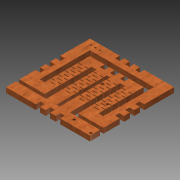
# Autodesk Inventor part: mech
Saved by Autodesk Inventor 2014 SP1 (Build 180222100, 222)
## iProperties
Created: 2015-02-17
Part Number: mech
Material: Wood (Cherry)
Document SubType Name: Modeling
Designer: Erin
Density: 0.63 g/cm^3
Appearance: Cherry - Natural Low Gloss
Author: Erin
Autodesk Inventor part; units mm, degrees
(part 1 of 2)
ref_plane "YZ Plane" through (0, 0, 0) normal (1, 0, 0) x (0, 1, 0)
ref_plane "XZ Plane" through (0, 0, 0) normal (0, 1, 0) x (-1, 0, 0)
ref_plane "XY Plane" through (0, 0, 0) normal (0, 0, 1) x (1, 0, 0)
sketch "slots" plane through (0, 0, 0) normal (0, 0, 1) x (1, 0, 0)
  line L0 (61.2067, 31.1821) -> (64.2567, 31.1821)
  line L1 (64.2567, 31.1821) -> (64.2567, 28.1071)
  line L2 (64.2567, 28.1071) -> (61.2067, 28.1071)
  line L3 (61.2067, 28.1071) -> (61.2067, 31.1821)
  line L4 (68.9317, 33.8834) -> (68.9317, 26.9198) construction
  line L5 (67.4067, 31.1821) -> (70.4567, 31.1821)
  line L6 (70.4567, 31.1821) -> (70.4567, 28.1071)
  line L7 (70.4567, 28.1071) -> (67.4067, 28.1071)
  line L8 (67.4067, 28.1071) -> (67.4067, 31.1821)
  line L9 (73.6067, 31.1821) -> (76.6567, 31.1821)
  line L10 (76.6567, 31.1821) -> (76.6567, 28.1071)
  line L11 (76.6567, 28.1071) -> (73.6067, 28.1071)
  line L12 (73.6067, 28.1071) -> (73.6067, 31.1821)
  line L13 (68.9317, 28.1071) -> (68.9317, 27.1937) construction
  point P0 (68.8645, 30.3856)
  dimension "d2" = 3.05
  dimension "d3" = 3.075
  dimension "d99" = 3.15
  dimension "d100" = 3.15
  measures "d2" distance of L1.end L2.end
  measures "d3" distance of L0.end L1.end
  measures "d99" distance between parallel lines of L8 L1
  measures "d100" distance between parallel lines of L12 L6
sketch "flexure" plane through (0, 0, 0) normal (0, 0, 1) x (1, 0, 0)
  line L0 (49.9032, 41.5133) -> (55.9032, 41.5133)
  line L1 (55.9032, 41.5133) -> (55.9032, 19.5133)
  line L2 (55.9032, 19.5133) -> (49.9032, 19.5133)
  line L3 (49.9032, 19.5133) -> (49.9032, 41.5133)
  line L4 (49.9032, 31.7633) -> (52.085, 31.7633)
  line L5 (52.085, 31.7633) -> (52.085, 31.2633)
  line L6 (52.085, 31.2633) -> (49.9032, 31.2633)
  line L7 (49.9032, 31.2633) -> (49.9032, 31.7633)
  line L8 (53.7214, 31.2633) -> (53.7214, 31.7633)
  line L9 (55.9032, 31.2633) -> (53.7214, 31.2633)
  line L10 (53.7214, 31.7633) -> (55.9032, 31.7633)
  line L11 (55.9032, 31.7633) -> (55.9032, 31.2633)
  line L12 (51.5395, 29.7633) -> (54.2668, 29.7633)
  line L13 (54.2668, 29.7633) -> (54.2668, 29.2633)
  line L14 (54.2668, 29.2633) -> (51.5395, 29.2633)
  line L15 (51.5395, 29.2633) -> (51.5395, 29.7633)
  line L16 (49.9032, 30.5133) -> (55.9032, 30.5133) construction
  line L17 (55.9032, 30.5133) -> (49.9032, 30.5133) construction
  line L18 (53.7214, 27.7633) -> (55.9032, 27.7633)
  line L19 (55.9032, 27.7633) -> (55.9032, 27.2633)
  line L20 (55.9032, 27.2633) -> (53.7214, 27.2633)
  line L21 (53.7214, 27.2633) -> (53.7214, 27.7633)
  line L22 (51.5395, 25.7633) -> (54.2668, 25.7633)
  line L23 (54.2668, 25.7633) -> (54.2668, 25.2633)
  line L24 (54.2668, 25.2633) -> (51.5395, 25.2633)
  line L25 (51.5395, 25.2633) -> (51.5395, 25.7633)
  line L26 (49.9032, 27.7633) -> (52.085, 27.7633)
  line L27 (52.085, 27.7633) -> (52.085, 27.2633)
  line L28 (52.085, 27.2633) -> (49.9032, 27.2633)
  line L29 (49.9032, 27.2633) -> (49.9032, 27.7633)
  line L30 (49.9032, 26.5133) -> (55.9032, 26.5133) construction
  line L31 (55.9032, 26.5133) -> (49.9032, 26.5133) construction
  line L32 (53.7214, 23.7633) -> (55.9032, 23.7633)
  line L33 (55.9032, 23.7633) -> (55.9032, 23.2633)
  line L34 (55.9032, 23.2633) -> (53.7214, 23.2633)
  line L35 (53.7214, 23.2633) -> (53.7214, 23.7633)
  line L36 (51.5395, 21.7633) -> (54.2668, 21.7633)
  line L37 (54.2668, 21.7633) -> (54.2668, 21.2633)
  line L38 (54.2668, 21.2633) -> (51.5395, 21.2633)
  line L39 (51.5395, 21.2633) -> (51.5395, 21.7633)
  line L40 (49.9032, 23.7633) -> (52.085, 23.7633)
  line L41 (52.085, 23.7633) -> (52.085, 23.2633)
  line L42 (52.085, 23.2633) -> (49.9032, 23.2633)
  line L43 (49.9032, 23.2633) -> (49.9032, 23.7633)
  line L44 (49.9032, 22.5133) -> (55.9032, 22.5133) construction
  line L45 (55.9032, 22.5133) -> (49.9032, 22.5133) construction
  line L46 (53.7214, 35.7633) -> (55.9032, 35.7633)
  line L47 (55.9032, 35.7633) -> (55.9032, 35.2633)
  line L48 (55.9032, 35.2633) -> (53.7214, 35.2633)
  line L49 (53.7214, 35.2633) -> (53.7214, 35.7633)
  line L50 (51.5395, 33.7633) -> (54.2668, 33.7633)
  line L51 (54.2668, 33.7633) -> (54.2668, 33.2633)
  line L52 (54.2668, 33.2633) -> (51.5395, 33.2633)
  line L53 (51.5395, 33.2633) -> (51.5395, 33.7633)
  line L54 (49.9032, 35.7633) -> (52.085, 35.7633)
  line L55 (52.085, 35.7633) -> (52.085, 35.2633)
  line L56 (52.085, 35.2633) -> (49.9032, 35.2633)
  line L57 (49.9032, 35.2633) -> (49.9032, 35.7633)
  line L58 (49.9032, 34.5133) -> (55.9032, 34.5133) construction
  line L59 (55.9032, 34.5133) -> (49.9032, 34.5133) construction
  line L60 (53.7214, 31.7633) -> (55.9032, 31.7633)
  line L61 (55.9032, 31.7633) -> (55.9032, 31.2633)
  line L62 (55.9032, 31.2633) -> (53.7214, 31.2633)
  line L63 (53.7214, 31.2633) -> (53.7214, 31.7633)
  line L64 (51.5395, 29.7633) -> (54.2668, 29.7633)
  line L65 (54.2668, 29.7633) -> (54.2668, 29.2633)
  line L66 (54.2668, 29.2633) -> (51.5395, 29.2633)
  line L67 (51.5395, 29.2633) -> (51.5395, 29.7633)
  line L68 (49.9032, 31.7633) -> (52.085, 31.7633)
  line L69 (52.085, 31.7633) -> (52.085, 31.2633)
  line L70 (52.085, 31.2633) -> (49.9032, 31.2633)
  line L71 (49.9032, 31.2633) -> (49.9032, 31.7633)
  line L72 (49.9032, 30.5133) -> (55.9032, 30.5133) construction
  line L73 (55.9032, 30.5133) -> (49.9032, 30.5133) construction
  line L74 (53.7214, 27.7633) -> (55.9032, 27.7633)
  line L75 (55.9032, 27.7633) -> (55.9032, 27.2633)
  line L76 (55.9032, 27.2633) -> (53.7214, 27.2633)
  line L77 (53.7214, 27.2633) -> (53.7214, 27.7633)
  line L78 (51.5395, 25.7633) -> (54.2668, 25.7633)
  line L79 (54.2668, 25.7633) -> (54.2668, 25.2633)
  line L80 (54.2668, 25.2633) -> (51.5395, 25.2633)
  line L81 (51.5395, 25.2633) -> (51.5395, 25.7633)
  line L82 (49.9032, 27.7633) -> (52.085, 27.7633)
  line L83 (52.085, 27.7633) -> (52.085, 27.2633)
  line L84 (52.085, 27.2633) -> (49.9032, 27.2633)
  line L85 (49.9032, 27.2633) -> (49.9032, 27.7633)
  line L86 (49.9032, 26.5133) -> (55.9032, 26.5133) construction
  line L87 (55.9032, 26.5133) -> (49.9032, 26.5133) construction
  line L88 (53.7214, 39.7633) -> (55.9032, 39.7633)
  line L89 (55.9032, 39.7633) -> (55.9032, 39.2633)
  line L90 (55.9032, 39.2633) -> (53.7214, 39.2633)
  line L91 (53.7214, 39.2633) -> (53.7214, 39.7633)
  line L92 (51.5395, 37.7633) -> (54.2668, 37.7633)
  line L93 (54.2668, 37.7633) -> (54.2668, 37.2633)
  line L94 (54.2668, 37.2633) -> (51.5395, 37.2633)
  line L95 (51.5395, 37.2633) -> (51.5395, 37.7633)
  line L96 (49.9032, 39.7633) -> (52.085, 39.7633)
  line L97 (52.085, 39.7633) -> (52.085, 39.2633)
  line L98 (52.085, 39.2633) -> (49.9032, 39.2633)
  line L99 (49.9032, 39.2633) -> (49.9032, 39.7633)
  line L100 (49.9032, 38.5133) -> (55.9032, 38.5133) construction
  line L101 (55.9032, 38.5133) -> (49.9032, 38.5133) construction
  line L102 (53.7214, 35.7633) -> (55.9032, 35.7633)
  line L103 (55.9032, 35.7633) -> (55.9032, 35.2633)
  line L104 (55.9032, 35.2633) -> (53.7214, 35.2633)
  line L105 (53.7214, 35.2633) -> (53.7214, 35.7633)
  line L106 (51.5395, 33.7633) -> (54.2668, 33.7633)
  line L107 (54.2668, 33.7633) -> (54.2668, 33.2633)
  line L108 (54.2668, 33.2633) -> (51.5395, 33.2633)
  line L109 (51.5395, 33.2633) -> (51.5395, 33.7633)
  line L110 (49.9032, 35.7633) -> (52.085, 35.7633)
  line L111 (52.085, 35.7633) -> (52.085, 35.2633)
  line L112 (52.085, 35.2633) -> (49.9032, 35.2633)
  line L113 (49.9032, 35.2633) -> (49.9032, 35.7633)
  line L114 (49.9032, 34.5133) -> (55.9032, 34.5133) construction
  line L115 (55.9032, 34.5133) -> (49.9032, 34.5133) construction
  line L116 (53.7214, 31.7633) -> (55.9032, 31.7633)
  line L117 (55.9032, 31.7633) -> (55.9032, 31.2633)
  line L118 (55.9032, 31.2633) -> (53.7214, 31.2633)
  line L119 (53.7214, 31.2633) -> (53.7214, 31.7633)
  line L120 (51.5395, 29.7633) -> (54.2668, 29.7633)
  line L121 (54.2668, 29.7633) -> (54.2668, 29.2633)
  line L122 (54.2668, 29.2633) -> (51.5395, 29.2633)
  line L123 (51.5395, 29.2633) -> (51.5395, 29.7633)
  line L124 (49.9032, 31.7633) -> (52.085, 31.7633)
  line L125 (52.085, 31.7633) -> (52.085, 31.2633)
  line L126 (52.085, 31.2633) -> (49.9032, 31.2633)
  line L127 (49.9032, 31.2633) -> (49.9032, 31.7633)
  line L128 (49.9032, 30.5133) -> (55.9032, 30.5133) construction
  line L129 (55.9032, 30.5133) -> (49.9032, 30.5133) construction
  line L130 (53.7214, 19.7633) -> (55.9032, 19.7633)
  line L131 (55.9032, 19.7633) -> (55.9032, 19.2633)
  line L132 (55.9032, 19.2633) -> (53.7214, 19.2633)
  line L133 (53.7214, 19.2633) -> (53.7214, 19.7633)
  line L134 (51.5395, 17.7633) -> (54.2668, 17.7633)
  line L135 (54.2668, 17.7633) -> (54.2668, 17.2633)
  line L136 (54.2668, 17.2633) -> (51.5395, 17.2633)
  line L137 (51.5395, 17.2633) -> (51.5395, 17.7633)
  line L138 (49.9032, 19.7633) -> (52.085, 19.7633)
  line L139 (52.085, 19.7633) -> (52.085, 19.2633)
  line L140 (52.085, 19.2633) -> (49.9032, 19.2633)
  line L141 (49.9032, 19.2633) -> (49.9032, 19.7633)
  line L142 (49.9032, 18.5133) -> (55.9032, 18.5133) construction
  line L143 (55.9032, 18.5133) -> (49.9032, 18.5133) construction
  line L144 (53.7214, 23.7633) -> (55.9032, 23.7633)
  line L145 (55.9032, 23.7633) -> (55.9032, 23.2633)
  line L146 (55.9032, 23.2633) -> (53.7214, 23.2633)
  line L147 (53.7214, 23.2633) -> (53.7214, 23.7633)
  line L148 (51.5395, 21.7633) -> (54.2668, 21.7633)
  line L149 (54.2668, 21.7633) -> (54.2668, 21.2633)
  line L150 (54.2668, 21.2633) -> (51.5395, 21.2633)
  line L151 (51.5395, 21.2633) -> (51.5395, 21.7633)
  line L152 (49.9032, 23.7633) -> (52.085, 23.7633)
  line L153 (52.085, 23.7633) -> (52.085, 23.2633)
  line L154 (52.085, 23.2633) -> (49.9032, 23.2633)
  line L155 (49.9032, 23.2633) -> (49.9032, 23.7633)
  line L156 (49.9032, 22.5133) -> (55.9032, 22.5133) construction
  line L157 (55.9032, 22.5133) -> (49.9032, 22.5133) construction
  line L158 (53.7214, 27.7633) -> (55.9032, 27.7633)
  line L159 (55.9032, 27.7633) -> (55.9032, 27.2633)
  line L160 (55.9032, 27.2633) -> (53.7214, 27.2633)
  line L161 (53.7214, 27.2633) -> (53.7214, 27.7633)
  line L162 (51.5395, 25.7633) -> (54.2668, 25.7633)
  line L163 (54.2668, 25.7633) -> (54.2668, 25.2633)
  line L164 (54.2668, 25.2633) -> (51.5395, 25.2633)
  line L165 (51.5395, 25.2633) -> (51.5395, 25.7633)
  line L166 (49.9032, 27.7633) -> (52.085, 27.7633)
  line L167 (52.085, 27.7633) -> (52.085, 27.2633)
  line L168 (52.085, 27.2633) -> (49.9032, 27.2633)
  line L169 (49.9032, 27.2633) -> (49.9032, 27.7633)
  line L170 (49.9032, 26.5133) -> (55.9032, 26.5133) construction
  line L171 (55.9032, 26.5133) -> (49.9032, 26.5133) construction
  line L172 (53.7214, 43.7633) -> (55.9032, 43.7633)
  line L173 (55.9032, 43.7633) -> (55.9032, 43.2633)
  line L174 (55.9032, 43.2633) -> (53.7214, 43.2633)
  line L175 (53.7214, 43.2633) -> (53.7214, 43.7633)
  line L176 (51.5395, 41.7633) -> (54.2668, 41.7633)
  line L177 (54.2668, 41.7633) -> (54.2668, 41.2633)
  line L178 (54.2668, 41.2633) -> (51.5395, 41.2633)
  line L179 (51.5395, 41.2633) -> (51.5395, 41.7633)
  line L180 (49.9032, 43.7633) -> (52.085, 43.7633)
  line L181 (52.085, 43.7633) -> (52.085, 43.2633)
  line L182 (52.085, 43.2633) -> (49.9032, 43.2633)
  line L183 (49.9032, 43.2633) -> (49.9032, 43.7633)
  line L184 (49.9032, 42.5133) -> (55.9032, 42.5133) construction
  line L185 (55.9032, 42.5133) -> (49.9032, 42.5133) construction
  line L186 (53.7214, 39.7633) -> (55.9032, 39.7633)
  line L187 (55.9032, 39.7633) -> (55.9032, 39.2633)
  line L188 (55.9032, 39.2633) -> (53.7214, 39.2633)
  line L189 (53.7214, 39.2633) -> (53.7214, 39.7633)
  line L190 (51.5395, 37.7633) -> (54.2668, 37.7633)
  line L191 (54.2668, 37.7633) -> (54.2668, 37.2633)
  line L192 (54.2668, 37.2633) -> (51.5395, 37.2633)
  line L193 (51.5395, 37.2633) -> (51.5395, 37.7633)
  line L194 (49.9032, 39.7633) -> (52.085, 39.7633)
  line L195 (52.085, 39.7633) -> (52.085, 39.2633)
  line L196 (52.085, 39.2633) -> (49.9032, 39.2633)
  line L197 (49.9032, 39.2633) -> (49.9032, 39.7633)
  line L198 (49.9032, 38.5133) -> (55.9032, 38.5133) construction
  line L199 (55.9032, 38.5133) -> (49.9032, 38.5133) construction
  line L200 (53.7214, 35.7633) -> (55.9032, 35.7633)
  line L201 (55.9032, 35.7633) -> (55.9032, 35.2633)
  line L202 (55.9032, 35.2633) -> (53.7214, 35.2633)
  line L203 (53.7214, 35.2633) -> (53.7214, 35.7633)
  line L204 (51.5395, 33.7633) -> (54.2668, 33.7633)
  line L205 (54.2668, 33.7633) -> (54.2668, 33.2633)
  line L206 (54.2668, 33.2633) -> (51.5395, 33.2633)
  line L207 (51.5395, 33.2633) -> (51.5395, 33.7633)
  line L208 (49.9032, 35.7633) -> (52.085, 35.7633)
  line L209 (52.085, 35.7633) -> (52.085, 35.2633)
  line L210 (52.085, 35.2633) -> (49.9032, 35.2633)
  line L211 (49.9032, 35.2633) -> (49.9032, 35.7633)
  line L212 (49.9032, 34.5133) -> (55.9032, 34.5133) construction
  line L213 (55.9032, 34.5133) -> (49.9032, 34.5133) construction
  line L214 (53.7214, 31.7633) -> (55.9032, 31.7633)
  line L215 (55.9032, 31.7633) -> (55.9032, 31.2633)
  line L216 (55.9032, 31.2633) -> (53.7214, 31.2633)
  line L217 (53.7214, 31.2633) -> (53.7214, 31.7633)
  line L218 (51.5395, 29.7633) -> (54.2668, 29.7633)
  line L219 (54.2668, 29.7633) -> (54.2668, 29.2633)
  line L220 (54.2668, 29.2633) -> (51.5395, 29.2633)
  line L221 (51.5395, 29.2633) -> (51.5395, 29.7633)
  line L222 (49.9032, 31.7633) -> (52.085, 31.7633)
  line L223 (52.085, 31.7633) -> (52.085, 31.2633)
  line L224 (52.085, 31.2633) -> (49.9032, 31.2633)
  line L225 (49.9032, 31.2633) -> (49.9032, 31.7633)
  line L226 (49.9032, 30.5133) -> (55.9032, 30.5133) construction
  line L227 (55.9032, 30.5133) -> (49.9032, 30.5133) construction
  point P0 (52.8239, 25.8216)
  dimension "d22" = 6
  dimension "d24" = 2.1818
  dimension "d27" = 3.8182
  dimension "d32" = 1.6364
  dimension "d33" = 2.7273
  dimension "d41" = 0.5
  dimension "d42" = 0.5
  dimension "d43" = 1.5
  dimension "d93" = 22
  dimension "d106" = 4
  dimension "d109" = 4
  dimension "d117" = 11.75
  measures "d22" distance of L1.end L2.end
  measures "d24" distance of L4.start L4.end
  measures "d27" distance of L6.end L9.end
  measures "d32" distance between parallel lines of L15 L3
  measures "d33" distance of L12.start L12.end
  measures "d41" distance of L4.end L5.end
  measures "d42" distance of L12.end L13.end
  measures "d43" distance between parallel lines of L12 L6
  measures "d93" distance of L0.end L1.end
  measures "d106" distance of L10.start L18.start
  measures "d109" distance of L10.start L46.start
  measures "d117" distance between parallel lines of L12 L0
sketch "Sketch1" plane through (0, 0, 0) normal (0, 0, 1) x (1, 0, 0)
  line L0 (-25, 25) -> (25, 25) construction
  line L1 (25, 25) -> (25, -25) construction
  line L2 (25, -25) -> (-25, -25) construction
  line L3 (-25, -25) -> (-25, 25) construction
  line L4 (-25, -25) -> (25, -25)
  line L5 (25, -25) -> (25, -19)
  line L6 (25, -19) -> (-25, -19)
  line L7 (-25, -19) -> (-25, -25)
  line L8 (0, 33.5916) -> (0, -39.9789) construction
  line L9 (-35.9054, 0) -> (42.6007, 0) construction
  line L10 (-25, 25) -> (25, 25)
  line L11 (25, 25) -> (25, 19)
  line L12 (25, 19) -> (-25, 19)
  line L13 (-25, 19) -> (-25, 25)
  line L14 (-25, 19) -> (-19, 19)
  line L15 (-19, 19) -> (-19, -17)
  line L16 (-19, -17) -> (-25, -17)
  line L17 (-25, -17) -> (-25, 19)
  line L18 (-19, -17) -> (-10, -17)
  line L19 (-10, -17) -> (-10, -11)
  line L20 (-10, -11) -> (-19, -11)
  line L21 (-19, -11) -> (-19, -17)
  line L22 (25, 19) -> (19, 19)
  line L23 (19, 19) -> (19, -17)
  line L24 (19, -17) -> (25, -17)
  line L25 (25, -17) -> (25, 19)
  line L26 (19, -17) -> (10, -17)
  line L27 (10, -17) -> (10, -11)
  line L28 (10, -11) -> (19, -11)
  line L29 (19, -11) -> (19, -17)
  line L30 (-16, 16) -> (16, 16)
  line L31 (16, 16) -> (16, 11)
  line L32 (16, 11) -> (-16, 11)
  line L33 (-16, 11) -> (-16, 16)
  line L34 (-7, -11) -> (-1, -11)
  line L35 (-1, -11) -> (-1, -19)
  line L36 (-1, -19) -> (-7, -19)
  line L37 (-7, -19) -> (-7, -11)
  line L38 (1, -11) -> (7, -11)
  line L39 (7, -11) -> (7, -19)
  line L40 (7, -19) -> (1, -19)
  line L41 (1, -19) -> (1, -11)
  line L42 (-68.1542, 16.5688) -> (-29.44, 16.5688) construction
  line L43 (-29.44, 16.5688) -> (-29.44, -5.0786) construction
  line L44 (-29.44, -5.0786) -> (-68.1542, -5.0786) construction
  line L45 (-68.1542, -5.0786) -> (-68.1542, 16.5688) construction
  circle A0 centre (-21.2866, 22) radius 0.5
  circle A1 centre (-18.6754, 22) radius 0.5
  circle A2 centre (-16, 22) radius 0.5
  line L46 (-7.725, 25) -> (-4.675, 25)
  line L47 (-4.675, 25) -> (-4.675, 21.925)
  line L48 (-4.675, 21.925) -> (-7.725, 21.925)
  line L49 (-7.725, 21.925) -> (-7.725, 25)
  line L50 (0, 27.7013) -> (0, 20.7377) construction
  line L51 (-1.525, 25) -> (1.525, 25)
  line L52 (1.525, 25) -> (1.525, 21.925)
  line L53 (1.525, 21.925) -> (-1.525, 21.925)
  line L54 (-1.525, 21.925) -> (-1.525, 25)
  line L55 (4.675, 25) -> (7.725, 25)
  line L56 (7.725, 25) -> (7.725, 21.925)
  line L57 (7.725, 21.925) -> (4.675, 21.925)
  line L58 (4.675, 21.925) -> (4.675, 25)
  line L59 (0, 21.925) -> (0, 21.0116) construction
  line L60 (-7.725, -21.925) -> (-4.675, -21.925)
  line L61 (-4.675, -21.925) -> (-4.675, -25)
  line L62 (-4.675, -25) -> (-7.725, -25)
  line L63 (-7.725, -25) -> (-7.725, -21.925)
  line L64 (0, -19.2237) -> (0, -26.1873) construction
  line L65 (-1.525, -21.925) -> (1.525, -21.925)
  line L66 (1.525, -21.925) -> (1.525, -25)
  line L67 (1.525, -25) -> (-1.525, -25)
  line L68 (-1.525, -25) -> (-1.525, -21.925)
  line L69 (4.675, -21.925) -> (7.725, -21.925)
  line L70 (7.725, -21.925) -> (7.725, -25)
  line L71 (7.725, -25) -> (4.675, -25)
  line L72 (4.675, -25) -> (4.675, -21.925)
  line L73 (0, -25) -> (0, -25.9134) construction
  line L74 (-25, -7.725) -> (-25, -4.675)
  line L75 (-25, -4.675) -> (-21.925, -4.675)
  line L76 (-21.925, -4.675) -> (-21.925, -7.725)
  line L77 (-21.925, -7.725) -> (-25, -7.725)
  line L78 (-27.7013, 0) -> (-20.7377, 0) construction
  line L79 (-25, -1.525) -> (-25, 1.525)
  line L80 (-25, 1.525) -> (-21.925, 1.525)
  line L81 (-21.925, 1.525) -> (-21.925, -1.525)
  line L82 (-21.925, -1.525) -> (-25, -1.525)
  line L83 (-25, 4.675) -> (-25, 7.725)
  line L84 (-25, 7.725) -> (-21.925, 7.725)
  line L85 (-21.925, 7.725) -> (-21.925, 4.675)
  line L86 (-21.925, 4.675) -> (-25, 4.675)
  line L87 (-21.925, 0) -> (-21.0116, 0) construction
  line L88 (21.925, -7.725) -> (21.925, -4.675)
  line L89 (21.925, -4.675) -> (25, -4.675)
  line L90 (25, -4.675) -> (25, -7.725)
  line L91 (25, -7.725) -> (21.925, -7.725)
  line L92 (19.2237, 0) -> (26.1873, 0) construction
  line L93 (21.925, -1.525) -> (21.925, 1.525)
  line L94 (21.925, 1.525) -> (25, 1.525)
  line L95 (25, 1.525) -> (25, -1.525)
  line L96 (25, -1.525) -> (21.925, -1.525)
  line L97 (21.925, 4.675) -> (21.925, 7.725)
  line L98 (21.925, 7.725) -> (25, 7.725)
  line L99 (25, 7.725) -> (25, 4.675)
  line L100 (25, 4.675) -> (21.925, 4.675)
  line L101 (25, 0) -> (25.9134, 0) construction
  line L102 (-16, 11) -> (-10, 11)
  line L103 (-10, 11) -> (-10, -11)
  line L104 (-10, -11) -> (-16, -11)
  line L105 (-16, -11) -> (-16, 11)
  line L106 (-16, 1.25) -> (-13.8182, 1.25)
  line L107 (-13.8182, 1.25) -> (-13.8182, 0.75)
  line L108 (-13.8182, 0.75) -> (-16, 0.75)
  line L109 (-16, 0.75) -> (-16, 1.25)
  line L110 (-12.1818, 0.75) -> (-12.1818, 1.25)
  line L111 (-10, 0.75) -> (-12.1818, 0.75)
  line L112 (-12.1818, 1.25) -> (-10, 1.25)
  line L113 (-10, 1.25) -> (-10, 0.75)
  line L114 (-14.3636, -0.75) -> (-11.6364, -0.75)
  line L115 (-11.6364, -0.75) -> (-11.6364, -1.25)
  line L116 (-11.6364, -1.25) -> (-14.3636, -1.25)
  line L117 (-14.3636, -1.25) -> (-14.3636, -0.75)
  line L118 (-16, 0) -> (-10, 0) construction
  line L119 (-10, 0) -> (-16, 0) construction
  line L120 (-12.1818, -2.75) -> (-10, -2.75)
  line L121 (-10, -2.75) -> (-10, -3.25)
  line L122 (-10, -3.25) -> (-12.1818, -3.25)
  line L123 (-12.1818, -3.25) -> (-12.1818, -2.75)
  line L124 (-14.3636, -4.75) -> (-11.6364, -4.75)
  line L125 (-11.6364, -4.75) -> (-11.6364, -5.25)
  line L126 (-11.6364, -5.25) -> (-14.3636, -5.25)
  line L127 (-14.3636, -5.25) -> (-14.3636, -4.75)
  line L128 (-16, -2.75) -> (-13.8182, -2.75)
  line L129 (-13.8182, -2.75) -> (-13.8182, -3.25)
  line L130 (-13.8182, -3.25) -> (-16, -3.25)
  line L131 (-16, -3.25) -> (-16, -2.75)
  line L132 (-16, -4) -> (-10, -4) construction
  line L133 (-10, -4) -> (-16, -4) construction
  line L134 (-12.1818, -6.75) -> (-10, -6.75)
  line L135 (-10, -6.75) -> (-10, -7.25)
  line L136 (-10, -7.25) -> (-12.1818, -7.25)
  line L137 (-12.1818, -7.25) -> (-12.1818, -6.75)
  line L138 (-14.3636, -8.75) -> (-11.6364, -8.75)
  line L139 (-11.6364, -8.75) -> (-11.6364, -9.25)
  line L140 (-11.6364, -9.25) -> (-14.3636, -9.25)
  line L141 (-14.3636, -9.25) -> (-14.3636, -8.75)
  line L142 (-16, -6.75) -> (-13.8182, -6.75)
  line L143 (-13.8182, -6.75) -> (-13.8182, -7.25)
  line L144 (-13.8182, -7.25) -> (-16, -7.25)
  line L145 (-16, -7.25) -> (-16, -6.75)
  line L146 (-16, -8) -> (-10, -8) construction
  line L147 (-10, -8) -> (-16, -8) construction
  line L148 (-12.1818, 5.25) -> (-10, 5.25)
  line L149 (-10, 5.25) -> (-10, 4.75)
  line L150 (-10, 4.75) -> (-12.1818, 4.75)
  line L151 (-12.1818, 4.75) -> (-12.1818, 5.25)
  line L152 (-14.3636, 3.25) -> (-11.6364, 3.25)
  line L153 (-11.6364, 3.25) -> (-11.6364, 2.75)
  line L154 (-11.6364, 2.75) -> (-14.3636, 2.75)
  line L155 (-14.3636, 2.75) -> (-14.3636, 3.25)
  line L156 (-16, 5.25) -> (-13.8182, 5.25)
  line L157 (-13.8182, 5.25) -> (-13.8182, 4.75)
  line L158 (-13.8182, 4.75) -> (-16, 4.75)
  line L159 (-16, 4.75) -> (-16, 5.25)
  line L160 (-16, 4) -> (-10, 4) construction
  line L161 (-10, 4) -> (-16, 4) construction
  line L162 (-12.1818, 1.25) -> (-10, 1.25)
  line L163 (-10, 1.25) -> (-10, 0.75)
  line L164 (-10, 0.75) -> (-12.1818, 0.75)
  line L165 (-12.1818, 0.75) -> (-12.1818, 1.25)
  line L166 (-14.3636, -0.75) -> (-11.6364, -0.75)
  line L167 (-11.6364, -0.75) -> (-11.6364, -1.25)
  line L168 (-11.6364, -1.25) -> (-14.3636, -1.25)
  line L169 (-14.3636, -1.25) -> (-14.3636, -0.75)
  line L170 (-16, 1.25) -> (-13.8182, 1.25)
  line L171 (-13.8182, 1.25) -> (-13.8182, 0.75)
  line L172 (-13.8182, 0.75) -> (-16, 0.75)
  line L173 (-16, 0.75) -> (-16, 1.25)
  line L174 (-16, 0) -> (-10, 0) construction
  line L175 (-10, 0) -> (-16, 0) construction
  line L176 (-12.1818, -2.75) -> (-10, -2.75)
  line L177 (-10, -2.75) -> (-10, -3.25)
  line L178 (-10, -3.25) -> (-12.1818, -3.25)
  line L179 (-12.1818, -3.25) -> (-12.1818, -2.75)
  line L180 (-14.3636, -4.75) -> (-11.6364, -4.75)
  line L181 (-11.6364, -4.75) -> (-11.6364, -5.25)
  line L182 (-11.6364, -5.25) -> (-14.3636, -5.25)
  line L183 (-14.3636, -5.25) -> (-14.3636, -4.75)
  line L184 (-16, -2.75) -> (-13.8182, -2.75)
  line L185 (-13.8182, -2.75) -> (-13.8182, -3.25)
  line L186 (-13.8182, -3.25) -> (-16, -3.25)
  line L187 (-16, -3.25) -> (-16, -2.75)
  line L188 (-16, -4) -> (-10, -4) construction
  line L189 (-10, -4) -> (-16, -4) construction
  line L190 (-12.1818, 9.25) -> (-10, 9.25)
  line L191 (-10, 9.25) -> (-10, 8.75)
  line L192 (-10, 8.75) -> (-12.1818, 8.75)
  line L193 (-12.1818, 8.75) -> (-12.1818, 9.25)
  line L194 (-14.3636, 7.25) -> (-11.6364, 7.25)
  line L195 (-11.6364, 7.25) -> (-11.6364, 6.75)
  line L196 (-11.6364, 6.75) -> (-14.3636, 6.75)
  line L197 (-14.3636, 6.75) -> (-14.3636, 7.25)
  line L198 (-16, 9.25) -> (-13.8182, 9.25)
  line L199 (-13.8182, 9.25) -> (-13.8182, 8.75)
  line L200 (-13.8182, 8.75) -> (-16, 8.75)
  line L201 (-16, 8.75) -> (-16, 9.25)
  line L202 (-16, 8) -> (-10, 8) construction
  line L203 (-10, 8) -> (-16, 8) construction
  line L204 (-12.1818, 5.25) -> (-10, 5.25)
  line L205 (-10, 5.25) -> (-10, 4.75)
  line L206 (-10, 4.75) -> (-12.1818, 4.75)
  line L207 (-12.1818, 4.75) -> (-12.1818, 5.25)
  line L208 (-14.3636, 3.25) -> (-11.6364, 3.25)
  line L209 (-11.6364, 3.25) -> (-11.6364, 2.75)
  line L210 (-11.6364, 2.75) -> (-14.3636, 2.75)
  line L211 (-14.3636, 2.75) -> (-14.3636, 3.25)
  line L212 (-16, 5.25) -> (-13.8182, 5.25)
  line L213 (-13.8182, 5.25) -> (-13.8182, 4.75)
  line L214 (-13.8182, 4.75) -> (-16, 4.75)
  line L215 (-16, 4.75) -> (-16, 5.25)
  line L216 (-16, 4) -> (-10, 4) construction
  line L217 (-10, 4) -> (-16, 4) construction
  line L218 (-12.1818, 1.25) -> (-10, 1.25)
  line L219 (-10, 1.25) -> (-10, 0.75)
  line L220 (-10, 0.75) -> (-12.1818, 0.75)
  line L221 (-12.1818, 0.75) -> (-12.1818, 1.25)
  line L222 (-14.3636, -0.75) -> (-11.6364, -0.75)
  line L223 (-11.6364, -0.75) -> (-11.6364, -1.25)
  line L224 (-11.6364, -1.25) -> (-14.3636, -1.25)
  line L225 (-14.3636, -1.25) -> (-14.3636, -0.75)
  line L226 (-16, 1.25) -> (-13.8182, 1.25)
  line L227 (-13.8182, 1.25) -> (-13.8182, 0.75)
  line L228 (-13.8182, 0.75) -> (-16, 0.75)
  line L229 (-16, 0.75) -> (-16, 1.25)
  line L230 (-16, 0) -> (-10, 0) construction
  line L231 (-10, 0) -> (-16, 0) construction
  line L232 (-12.1818, -10.75) -> (-10, -10.75)
  line L233 (-10, -10.75) -> (-10, -11.25)
  line L234 (-10, -11.25) -> (-12.1818, -11.25)
  line L235 (-12.1818, -11.25) -> (-12.1818, -10.75)
  line L236 (-14.3636, -12.75) -> (-11.6364, -12.75)
  line L237 (-11.6364, -12.75) -> (-11.6364, -13.25)
  line L238 (-11.6364, -13.25) -> (-14.3636, -13.25)
  line L239 (-14.3636, -13.25) -> (-14.3636, -12.75)
  line L240 (-16, -10.75) -> (-13.8182, -10.75)
  line L241 (-13.8182, -10.75) -> (-13.8182, -11.25)
  line L242 (-13.8182, -11.25) -> (-16, -11.25)
  line L243 (-16, -11.25) -> (-16, -10.75)
  line L244 (-16, -12) -> (-10, -12) construction
  line L245 (-10, -12) -> (-16, -12) construction
  line L246 (-12.1818, -6.75) -> (-10, -6.75)
  line L247 (-10, -6.75) -> (-10, -7.25)
  line L248 (-10, -7.25) -> (-12.1818, -7.25)
  line L249 (-12.1818, -7.25) -> (-12.1818, -6.75)
  line L250 (-14.3636, -8.75) -> (-11.6364, -8.75)
  line L251 (-11.6364, -8.75) -> (-11.6364, -9.25)
  line L252 (-11.6364, -9.25) -> (-14.3636, -9.25)
  line L253 (-14.3636, -9.25) -> (-14.3636, -8.75)
  line L254 (-16, -6.75) -> (-13.8182, -6.75)
  line L255 (-13.8182, -6.75) -> (-13.8182, -7.25)
  line L256 (-13.8182, -7.25) -> (-16, -7.25)
  line L257 (-16, -7.25) -> (-16, -6.75)
  line L258 (-16, -8) -> (-10, -8) construction
  line L259 (-10, -8) -> (-16, -8) construction
  line L260 (-12.1818, -2.75) -> (-10, -2.75)
  line L261 (-10, -2.75) -> (-10, -3.25)
  line L262 (-10, -3.25) -> (-12.1818, -3.25)
  line L263 (-12.1818, -3.25) -> (-12.1818, -2.75)
  line L264 (-14.3636, -4.75) -> (-11.6364, -4.75)
  line L265 (-11.6364, -4.75) -> (-11.6364, -5.25)
  line L266 (-11.6364, -5.25) -> (-14.3636, -5.25)
  line L267 (-14.3636, -5.25) -> (-14.3636, -4.75)
  line L268 (-16, -2.75) -> (-13.8182, -2.75)
  line L269 (-13.8182, -2.75) -> (-13.8182, -3.25)
  line L270 (-13.8182, -3.25) -> (-16, -3.25)
  line L271 (-16, -3.25) -> (-16, -2.75)
  line L272 (-16, -4) -> (-10, -4) construction
  line L273 (-10, -4) -> (-16, -4) construction
  line L274 (-12.1818, 13.25) -> (-10, 13.25)
  line L275 (-10, 13.25) -> (-10, 12.75)
  line L276 (-10, 12.75) -> (-12.1818, 12.75)
  line L277 (-12.1818, 12.75) -> (-12.1818, 13.25)
  line L278 (-14.3636, 11.25) -> (-11.6364, 11.25)
  line L279 (-11.6364, 11.25) -> (-11.6364, 10.75)
  line L280 (-11.6364, 10.75) -> (-14.3636, 10.75)
  line L281 (-14.3636, 10.75) -> (-14.3636, 11.25)
  line L282 (-16, 13.25) -> (-13.8182, 13.25)
  line L283 (-13.8182, 13.25) -> (-13.8182, 12.75)
  line L284 (-13.8182, 12.75) -> (-16, 12.75)
  line L285 (-16, 12.75) -> (-16, 13.25)
  line L286 (-16, 12) -> (-10, 12) construction
  line L287 (-10, 12) -> (-16, 12) construction
  line L288 (-12.1818, 9.25) -> (-10, 9.25)
  line L289 (-10, 9.25) -> (-10, 8.75)
  line L290 (-10, 8.75) -> (-12.1818, 8.75)
  line L291 (-12.1818, 8.75) -> (-12.1818, 9.25)
  line L292 (-14.3636, 7.25) -> (-11.6364, 7.25)
  line L293 (-11.6364, 7.25) -> (-11.6364, 6.75)
  line L294 (-11.6364, 6.75) -> (-14.3636, 6.75)
  line L295 (-14.3636, 6.75) -> (-14.3636, 7.25)
  line L296 (-16, 9.25) -> (-13.8182, 9.25)
  line L297 (-13.8182, 9.25) -> (-13.8182, 8.75)
  line L298 (-13.8182, 8.75) -> (-16, 8.75)
  line L299 (-16, 8.75) -> (-16, 9.25)
  line L300 (-16, 8) -> (-10, 8) construction
  line L301 (-10, 8) -> (-16, 8) construction
  line L302 (-12.1818, 5.25) -> (-10, 5.25)
  line L303 (-10, 5.25) -> (-10, 4.75)
  line L304 (-10, 4.75) -> (-12.1818, 4.75)
  line L305 (-12.1818, 4.75) -> (-12.1818, 5.25)
  line L306 (-14.3636, 3.25) -> (-11.6364, 3.25)
  line L307 (-11.6364, 3.25) -> (-11.6364, 2.75)
  line L308 (-11.6364, 2.75) -> (-14.3636, 2.75)
  line L309 (-14.3636, 2.75) -> (-14.3636, 3.25)
  line L310 (-16, 5.25) -> (-13.8182, 5.25)
  line L311 (-13.8182, 5.25) -> (-13.8182, 4.75)
  line L312 (-13.8182, 4.75) -> (-16, 4.75)
  line L313 (-16, 4.75) -> (-16, 5.25)
  line L314 (-16, 4) -> (-10, 4) construction
  line L315 (-10, 4) -> (-16, 4) construction
  line L316 (-12.1818, 1.25) -> (-10, 1.25)
  line L317 (-10, 1.25) -> (-10, 0.75)
  line L318 (-10, 0.75) -> (-12.1818, 0.75)
  line L319 (-12.1818, 0.75) -> (-12.1818, 1.25)
  line L320 (-14.3636, -0.75) -> (-11.6364, -0.75)
  line L321 (-11.6364, -0.75) -> (-11.6364, -1.25)
  line L322 (-11.6364, -1.25) -> (-14.3636, -1.25)
  line L323 (-14.3636, -1.25) -> (-14.3636, -0.75)
  line L324 (-16, 1.25) -> (-13.8182, 1.25)
  line L325 (-13.8182, 1.25) -> (-13.8182, 0.75)
  line L326 (-13.8182, 0.75) -> (-16, 0.75)
  line L327 (-16, 0.75) -> (-16, 1.25)
  line L328 (-16, 0) -> (-10, 0) construction
  line L329 (-10, 0) -> (-16, 0) construction
  line L330 (10, 11) -> (16, 11)
  line L331 (16, 11) -> (16, -11)
  line L332 (16, -11) -> (10, -11)
  line L333 (10, -11) -> (10, 11)
  line L334 (10, 1.25) -> (12.1818, 1.25)
  line L335 (12.1818, 1.25) -> (12.1818, 0.75)
  line L336 (12.1818, 0.75) -> (10, 0.75)
  line L337 (10, 0.75) -> (10, 1.25)
  line L338 (13.8182, 0.75) -> (13.8182, 1.25)
  line L339 (16, 0.75) -> (13.8182, 0.75)
  line L340 (13.8182, 1.25) -> (16, 1.25)
  line L341 (16, 1.25) -> (16, 0.75)
  line L342 (11.6364, -0.75) -> (14.3636, -0.75)
  line L343 (14.3636, -0.75) -> (14.3636, -1.25)
  line L344 (14.3636, -1.25) -> (11.6364, -1.25)
  line L345 (11.6364, -1.25) -> (11.6364, -0.75)
  line L346 (10, 0) -> (16, 0) construction
  line L347 (16, 0) -> (10, 0) construction
  line L348 (13.8182, -2.75) -> (16, -2.75)
  line L349 (16, -2.75) -> (16, -3.25)
  line L350 (16, -3.25) -> (13.8182, -3.25)
  line L351 (13.8182, -3.25) -> (13.8182, -2.75)
  line L352 (11.6364, -4.75) -> (14.3636, -4.75)
  line L353 (14.3636, -4.75) -> (14.3636, -5.25)
  line L354 (14.3636, -5.25) -> (11.6364, -5.25)
  line L355 (11.6364, -5.25) -> (11.6364, -4.75)
  line L356 (10, -2.75) -> (12.1818, -2.75)
  line L357 (12.1818, -2.75) -> (12.1818, -3.25)
  line L358 (12.1818, -3.25) -> (10, -3.25)
  line L359 (10, -3.25) -> (10, -2.75)
  line L360 (10, -4) -> (16, -4) construction
  line L361 (16, -4) -> (10, -4) construction
  line L362 (13.8182, -6.75) -> (16, -6.75)
  line L363 (16, -6.75) -> (16, -7.25)
  line L364 (16, -7.25) -> (13.8182, -7.25)
  line L365 (13.8182, -7.25) -> (13.8182, -6.75)
  line L366 (11.6364, -8.75) -> (14.3636, -8.75)
  line L367 (14.3636, -8.75) -> (14.3636, -9.25)
  line L368 (14.3636, -9.25) -> (11.6364, -9.25)
  line L369 (11.6364, -9.25) -> (11.6364, -8.75)
  line L370 (10, -6.75) -> (12.1818, -6.75)
  line L371 (12.1818, -6.75) -> (12.1818, -7.25)
  line L372 (12.1818, -7.25) -> (10, -7.25)
  line L373 (10, -7.25) -> (10, -6.75)
  line L374 (10, -8) -> (16, -8) construction
  line L375 (16, -8) -> (10, -8) construction
  line L376 (13.8182, 5.25) -> (16, 5.25)
  line L377 (16, 5.25) -> (16, 4.75)
  line L378 (16, 4.75) -> (13.8182, 4.75)
  line L379 (13.8182, 4.75) -> (13.8182, 5.25)
  line L380 (11.6364, 3.25) -> (14.3636, 3.25)
  line L381 (14.3636, 3.25) -> (14.3636, 2.75)
  line L382 (14.3636, 2.75) -> (11.6364, 2.75)
  line L383 (11.6364, 2.75) -> (11.6364, 3.25)
  line L384 (10, 5.25) -> (12.1818, 5.25)
  line L385 (12.1818, 5.25) -> (12.1818, 4.75)
  line L386 (12.1818, 4.75) -> (10, 4.75)
  line L387 (10, 4.75) -> (10, 5.25)
  line L388 (10, 4) -> (16, 4) construction
  line L389 (16, 4) -> (10, 4) construction
  line L390 (13.8182, 1.25) -> (16, 1.25)
  line L391 (16, 1.25) -> (16, 0.75)
  line L392 (16, 0.75) -> (13.8182, 0.75)
  line L393 (13.8182, 0.75) -> (13.8182, 1.25)
  line L394 (11.6364, -0.75) -> (14.3636, -0.75)
  line L395 (14.3636, -0.75) -> (14.3636, -1.25)
  line L396 (14.3636, -1.25) -> (11.6364, -1.25)
  line L397 (11.6364, -1.25) -> (11.6364, -0.75)
  line L398 (10, 1.25) -> (12.1818, 1.25)
  line L399 (12.1818, 1.25) -> (12.1818, 0.75)
  line L400 (12.1818, 0.75) -> (10, 0.75)
  line L401 (10, 0.75) -> (10, 1.25)
  line L402 (10, 0) -> (16, 0) construction
  line L403 (16, 0) -> (10, 0) construction
  line L404 (13.8182, -2.75) -> (16, -2.75)
  line L405 (16, -2.75) -> (16, -3.25)
  line L406 (16, -3.25) -> (13.8182, -3.25)
  line L407 (13.8182, -3.25) -> (13.8182, -2.75)
  line L408 (11.6364, -4.75) -> (14.3636, -4.75)
  line L409 (14.3636, -4.75) -> (14.3636, -5.25)
  line L410 (14.3636, -5.25) -> (11.6364, -5.25)
  line L411 (11.6364, -5.25) -> (11.6364, -4.75)
  line L412 (10, -2.75) -> (12.1818, -2.75)
  line L413 (12.1818, -2.75) -> (12.1818, -3.25)
  line L414 (12.1818, -3.25) -> (10, -3.25)
  line L415 (10, -3.25) -> (10, -2.75)
  line L416 (10, -4) -> (16, -4) construction
  line L417 (16, -4) -> (10, -4) construction
  line L418 (13.8182, 9.25) -> (16, 9.25)
  line L419 (16, 9.25) -> (16, 8.75)
  line L420 (16, 8.75) -> (13.8182, 8.75)
  line L421 (13.8182, 8.75) -> (13.8182, 9.25)
  line L422 (11.6364, 7.25) -> (14.3636, 7.25)
  line L423 (14.3636, 7.25) -> (14.3636, 6.75)
  line L424 (14.3636, 6.75) -> (11.6364, 6.75)
  line L425 (11.6364, 6.75) -> (11.6364, 7.25)
  line L426 (10, 9.25) -> (12.1818, 9.25)
  line L427 (12.1818, 9.25) -> (12.1818, 8.75)
  line L428 (12.1818, 8.75) -> (10, 8.75)
  line L429 (10, 8.75) -> (10, 9.25)
  line L430 (10, 8) -> (16, 8) construction
  line L431 (16, 8) -> (10, 8) construction
  line L432 (13.8182, 5.25) -> (16, 5.25)
  line L433 (16, 5.25) -> (16, 4.75)
  line L434 (16, 4.75) -> (13.8182, 4.75)
  line L435 (13.8182, 4.75) -> (13.8182, 5.25)
  line L436 (11.6364, 3.25) -> (14.3636, 3.25)
  line L437 (14.3636, 3.25) -> (14.3636, 2.75)
  line L438 (14.3636, 2.75) -> (11.6364, 2.75)
  line L439 (11.6364, 2.75) -> (11.6364, 3.25)
  line L440 (10, 5.25) -> (12.1818, 5.25)
  line L441 (12.1818, 5.25) -> (12.1818, 4.75)
  line L442 (12.1818, 4.75) -> (10, 4.75)
  line L443 (10, 4.75) -> (10, 5.25)
  line L444 (10, 4) -> (16, 4) construction
  line L445 (16, 4) -> (10, 4) construction
  line L446 (13.8182, 1.25) -> (16, 1.25)
  line L447 (16, 1.25) -> (16, 0.75)
  line L448 (16, 0.75) -> (13.8182, 0.75)
  line L449 (13.8182, 0.75) -> (13.8182, 1.25)
  line L450 (11.6364, -0.75) -> (14.3636, -0.75)
  line L451 (14.3636, -0.75) -> (14.3636, -1.25)
  line L452 (14.3636, -1.25) -> (11.6364, -1.25)
  line L453 (11.6364, -1.25) -> (11.6364, -0.75)
  line L454 (10, 1.25) -> (12.1818, 1.25)
  line L455 (12.1818, 1.25) -> (12.1818, 0.75)
  line L456 (12.1818, 0.75) -> (10, 0.75)
  line L457 (10, 0.75) -> (10, 1.25)
  line L458 (10, 0) -> (16, 0) construction
  line L459 (16, 0) -> (10, 0) construction
  line L460 (13.8182, -10.75) -> (16, -10.75)
  line L461 (16, -10.75) -> (16, -11.25)
  line L462 (16, -11.25) -> (13.8182, -11.25)
  line L463 (13.8182, -11.25) -> (13.8182, -10.75)
  line L464 (11.6364, -12.75) -> (14.3636, -12.75)
  line L465 (14.3636, -12.75) -> (14.3636, -13.25)
  line L466 (14.3636, -13.25) -> (11.6364, -13.25)
  line L467 (11.6364, -13.25) -> (11.6364, -12.75)
  line L468 (10, -10.75) -> (12.1818, -10.75)
  line L469 (12.1818, -10.75) -> (12.1818, -11.25)
  line L470 (12.1818, -11.25) -> (10, -11.25)
  line L471 (10, -11.25) -> (10, -10.75)
  line L472 (10, -12) -> (16, -12) construction
  line L473 (16, -12) -> (10, -12) construction
  line L474 (13.8182, -6.75) -> (16, -6.75)
  line L475 (16, -6.75) -> (16, -7.25)
  line L476 (16, -7.25) -> (13.8182, -7.25)
  line L477 (13.8182, -7.25) -> (13.8182, -6.75)
  line L478 (11.6364, -8.75) -> (14.3636, -8.75)
  line L479 (14.3636, -8.75) -> (14.3636, -9.25)
  line L480 (14.3636, -9.25) -> (11.6364, -9.25)
  line L481 (11.6364, -9.25) -> (11.6364, -8.75)
  line L482 (10, -6.75) -> (12.1818, -6.75)
  line L483 (12.1818, -6.75) -> (12.1818, -7.25)
  line L484 (12.1818, -7.25) -> (10, -7.25)
  line L485 (10, -7.25) -> (10, -6.75)
  line L486 (10, -8) -> (16, -8) construction
  line L487 (16, -8) -> (10, -8) construction
  line L488 (13.8182, -2.75) -> (16, -2.75)
  line L489 (16, -2.75) -> (16, -3.25)
  line L490 (16, -3.25) -> (13.8182, -3.25)
  line L491 (13.8182, -3.25) -> (13.8182, -2.75)
  line L492 (11.6364, -4.75) -> (14.3636, -4.75)
  line L493 (14.3636, -4.75) -> (14.3636, -5.25)
  line L494 (14.3636, -5.25) -> (11.6364, -5.25)
  line L495 (11.6364, -5.25) -> (11.6364, -4.75)
  line L496 (10, -2.75) -> (12.1818, -2.75)
  line L497 (12.1818, -2.75) -> (12.1818, -3.25)
  line L498 (12.1818, -3.25) -> (10, -3.25)
  line L499 (10, -3.25) -> (10, -2.75)
  line L500 (10, -4) -> (16, -4) construction
  line L501 (16, -4) -> (10, -4) construction
  line L502 (13.8182, 13.25) -> (16, 13.25)
  line L503 (16, 13.25) -> (16, 12.75)
  line L504 (16, 12.75) -> (13.8182, 12.75)
  line L505 (13.8182, 12.75) -> (13.8182, 13.25)
  line L506 (11.6364, 11.25) -> (14.3636, 11.25)
  line L507 (14.3636, 11.25) -> (14.3636, 10.75)
  line L508 (14.3636, 10.75) -> (11.6364, 10.75)
  line L509 (11.6364, 10.75) -> (11.6364, 11.25)
  line L510 (10, 13.25) -> (12.1818, 13.25)
  line L511 (12.1818, 13.25) -> (12.1818, 12.75)
  line L512 (12.1818, 12.75) -> (10, 12.75)
  line L513 (10, 12.75) -> (10, 13.25)
  line L514 (10, 12) -> (16, 12) construction
  line L515 (16, 12) -> (10, 12) construction
  line L516 (13.8182, 9.25) -> (16, 9.25)
  line L517 (16, 9.25) -> (16, 8.75)
  line L518 (16, 8.75) -> (13.8182, 8.75)
  line L519 (13.8182, 8.75) -> (13.8182, 9.25)
  line L520 (11.6364, 7.25) -> (14.3636, 7.25)
  line L521 (14.3636, 7.25) -> (14.3636, 6.75)
  line L522 (14.3636, 6.75) -> (11.6364, 6.75)
  line L523 (11.6364, 6.75) -> (11.6364, 7.25)
  line L524 (10, 9.25) -> (12.1818, 9.25)
  line L525 (12.1818, 9.25) -> (12.1818, 8.75)
  line L526 (12.1818, 8.75) -> (10, 8.75)
  line L527 (10, 8.75) -> (10, 9.25)
  line L528 (10, 8) -> (16, 8) construction
  line L529 (16, 8) -> (10, 8) construction
  line L530 (13.8182, 5.25) -> (16, 5.25)
  line L531 (16, 5.25) -> (16, 4.75)
  line L532 (16, 4.75) -> (13.8182, 4.75)
  line L533 (13.8182, 4.75) -> (13.8182, 5.25)
  line L534 (11.6364, 3.25) -> (14.3636, 3.25)
  line L535 (14.3636, 3.25) -> (14.3636, 2.75)
  line L536 (14.3636, 2.75) -> (11.6364, 2.75)
  line L537 (11.6364, 2.75) -> (11.6364, 3.25)
  line L538 (10, 5.25) -> (12.1818, 5.25)
  line L539 (12.1818, 5.25) -> (12.1818, 4.75)
  line L540 (12.1818, 4.75) -> (10, 4.75)
  line L541 (10, 4.75) -> (10, 5.25)
  line L542 (10, 4) -> (16, 4) construction
  line L543 (16, 4) -> (10, 4) construction
  line L544 (13.8182, 1.25) -> (16, 1.25)
  line L545 (16, 1.25) -> (16, 0.75)
  line L546 (16, 0.75) -> (13.8182, 0.75)
  line L547 (13.8182, 0.75) -> (13.8182, 1.25)
  line L548 (11.6364, -0.75) -> (14.3636, -0.75)
  line L549 (14.3636, -0.75) -> (14.3636, -1.25)
  line L550 (14.3636, -1.25) -> (11.6364, -1.25)
  line L551 (11.6364, -1.25) -> (11.6364, -0.75)
  line L552 (10, 1.25) -> (12.1818, 1.25)
  line L553 (12.1818, 1.25) -> (12.1818, 0.75)
  line L554 (12.1818, 0.75) -> (10, 0.75)
  line L555 (10, 0.75) -> (10, 1.25)
  line L556 (10, 0) -> (16, 0) construction
  line L557 (16, 0) -> (10, 0) construction
  line L558 (1, 11) -> (7, 11)
  line L559 (7, 11) -> (7, -11)
  line L560 (7, -11) -> (1, -11)
  line L561 (1, -11) -> (1, 11)
  line L562 (1, 1.25) -> (3.1818, 1.25)
  line L563 (3.1818, 1.25) -> (3.1818, 0.75)
  line L564 (3.1818, 0.75) -> (1, 0.75)
  line L565 (1, 0.75) -> (1, 1.25)
  line L566 (4.8182, 0.75) -> (4.8182, 1.25)
  line L567 (7, 0.75) -> (4.8182, 0.75)
  line L568 (4.8182, 1.25) -> (7, 1.25)
  line L569 (7, 1.25) -> (7, 0.75)
  line L570 (2.6364, -0.75) -> (5.3636, -0.75)
  line L571 (5.3636, -0.75) -> (5.3636, -1.25)
  line L572 (5.3636, -1.25) -> (2.6364, -1.25)
  line L573 (2.6364, -1.25) -> (2.6364, -0.75)
  line L574 (1, 0) -> (7, 0) construction
  line L575 (7, 0) -> (1, 0) construction
  line L576 (4.8182, -2.75) -> (7, -2.75)
  line L577 (7, -2.75) -> (7, -3.25)
  line L578 (7, -3.25) -> (4.8182, -3.25)
  line L579 (4.8182, -3.25) -> (4.8182, -2.75)
  line L580 (2.6364, -4.75) -> (5.3636, -4.75)
  line L581 (5.3636, -4.75) -> (5.3636, -5.25)
  line L582 (5.3636, -5.25) -> (2.6364, -5.25)
  line L583 (2.6364, -5.25) -> (2.6364, -4.75)
  line L584 (1, -2.75) -> (3.1818, -2.75)
  line L585 (3.1818, -2.75) -> (3.1818, -3.25)
  line L586 (3.1818, -3.25) -> (1, -3.25)
  line L587 (1, -3.25) -> (1, -2.75)
  line L588 (1, -4) -> (7, -4) construction
  line L589 (7, -4) -> (1, -4) construction
  line L590 (4.8182, -6.75) -> (7, -6.75)
  line L591 (7, -6.75) -> (7, -7.25)
  line L592 (7, -7.25) -> (4.8182, -7.25)
  line L593 (4.8182, -7.25) -> (4.8182, -6.75)
  line L594 (2.6364, -8.75) -> (5.3636, -8.75)
  line L595 (5.3636, -8.75) -> (5.3636, -9.25)
  line L596 (5.3636, -9.25) -> (2.6364, -9.25)
  line L597 (2.6364, -9.25) -> (2.6364, -8.75)
  line L598 (1, -6.75) -> (3.1818, -6.75)
  line L599 (3.1818, -6.75) -> (3.1818, -7.25)
  line L600 (3.1818, -7.25) -> (1, -7.25)
  line L601 (1, -7.25) -> (1, -6.75)
  line L602 (1, -8) -> (7, -8) construction
  line L603 (7, -8) -> (1, -8) construction
  line L604 (4.8182, 5.25) -> (7, 5.25)
  line L605 (7, 5.25) -> (7, 4.75)
  line L606 (7, 4.75) -> (4.8182, 4.75)
  line L607 (4.8182, 4.75) -> (4.8182, 5.25)
  line L608 (2.6364, 3.25) -> (5.3636, 3.25)
  line L609 (5.3636, 3.25) -> (5.3636, 2.75)
  line L610 (5.3636, 2.75) -> (2.6364, 2.75)
  line L611 (2.6364, 2.75) -> (2.6364, 3.25)
  line L612 (1, 5.25) -> (3.1818, 5.25)
  line L613 (3.1818, 5.25) -> (3.1818, 4.75)
  line L614 (3.1818, 4.75) -> (1, 4.75)
  line L615 (1, 4.75) -> (1, 5.25)
  line L616 (1, 4) -> (7, 4) construction
  line L617 (7, 4) -> (1, 4) construction
  line L618 (4.8182, 1.25) -> (7, 1.25)
  line L619 (7, 1.25) -> (7, 0.75)
  line L620 (7, 0.75) -> (4.8182, 0.75)
  line L621 (4.8182, 0.75) -> (4.8182, 1.25)
  line L622 (2.6364, -0.75) -> (5.3636, -0.75)
  line L623 (5.3636, -0.75) -> (5.3636, -1.25)
  line L624 (5.3636, -1.25) -> (2.6364, -1.25)
  line L625 (2.6364, -1.25) -> (2.6364, -0.75)
  line L626 (1, 1.25) -> (3.1818, 1.25)
  line L627 (3.1818, 1.25) -> (3.1818, 0.75)
  line L628 (3.1818, 0.75) -> (1, 0.75)
  line L629 (1, 0.75) -> (1, 1.25)
  line L630 (1, 0) -> (7, 0) construction
  line L631 (7, 0) -> (1, 0) construction
  line L632 (4.8182, -2.75) -> (7, -2.75)
  line L633 (7, -2.75) -> (7, -3.25)
  line L634 (7, -3.25) -> (4.8182, -3.25)
  line L635 (4.8182, -3.25) -> (4.8182, -2.75)
  line L636 (2.6364, -4.75) -> (5.3636, -4.75)
  line L637 (5.3636, -4.75) -> (5.3636, -5.25)
  line L638 (5.3636, -5.25) -> (2.6364, -5.25)
  line L639 (2.6364, -5.25) -> (2.6364, -4.75)
  line L640 (1, -2.75) -> (3.1818, -2.75)
  line L641 (3.1818, -2.75) -> (3.1818, -3.25)
  line L642 (3.1818, -3.25) -> (1, -3.25)
  line L643 (1, -3.25) -> (1, -2.75)
  line L644 (1, -4) -> (7, -4) construction
  line L645 (7, -4) -> (1, -4) construction
  line L646 (4.8182, 9.25) -> (7, 9.25)
  line L647 (7, 9.25) -> (7, 8.75)
  line L648 (7, 8.75) -> (4.8182, 8.75)
  line L649 (4.8182, 8.75) -> (4.8182, 9.25)
  line L650 (2.6364, 7.25) -> (5.3636, 7.25)
  line L651 (5.3636, 7.25) -> (5.3636, 6.75)
  line L652 (5.3636, 6.75) -> (2.6364, 6.75)
  line L653 (2.6364, 6.75) -> (2.6364, 7.25)
  line L654 (1, 9.25) -> (3.1818, 9.25)
  line L655 (3.1818, 9.25) -> (3.1818, 8.75)
  line L656 (3.1818, 8.75) -> (1, 8.75)
  line L657 (1, 8.75) -> (1, 9.25)
  line L658 (1, 8) -> (7, 8) construction
  line L659 (7, 8) -> (1, 8) construction
  line L660 (4.8182, 5.25) -> (7, 5.25)
  line L661 (7, 5.25) -> (7, 4.75)
  line L662 (7, 4.75) -> (4.8182, 4.75)
  line L663 (4.8182, 4.75) -> (4.8182, 5.25)
  line L664 (2.6364, 3.25) -> (5.3636, 3.25)
  line L665 (5.3636, 3.25) -> (5.3636, 2.75)
  line L666 (5.3636, 2.75) -> (2.6364, 2.75)
  line L667 (2.6364, 2.75) -> (2.6364, 3.25)
  line L668 (1, 5.25) -> (3.1818, 5.25)
  line L669 (3.1818, 5.25) -> (3.1818, 4.75)
  line L670 (3.1818, 4.75) -> (1, 4.75)
  line L671 (1, 4.75) -> (1, 5.25)
  line L672 (1, 4) -> (7, 4) construction
  line L673 (7, 4) -> (1, 4) construction
  line L674 (4.8182, 1.25) -> (7, 1.25)
  line L675 (7, 1.25) -> (7, 0.75)
  line L676 (7, 0.75) -> (4.8182, 0.75)
  line L677 (4.8182, 0.75) -> (4.8182, 1.25)
  line L678 (2.6364, -0.75) -> (5.3636, -0.75)
  line L679 (5.3636, -0.75) -> (5.3636, -1.25)
  line L680 (5.3636, -1.25) -> (2.6364, -1.25)
  line L681 (2.6364, -1.25) -> (2.6364, -0.75)
  line L682 (1, 1.25) -> (3.1818, 1.25)
  line L683 (3.1818, 1.25) -> (3.1818, 0.75)
  line L684 (3.1818, 0.75) -> (1, 0.75)
  line L685 (1, 0.75) -> (1, 1.25)
  line L686 (1, 0) -> (7, 0) construction
  line L687 (7, 0) -> (1, 0) construction
  line L688 (4.8182, -10.75) -> (7, -10.75)
  line L689 (7, -10.75) -> (7, -11.25)
  line L690 (7, -11.25) -> (4.8182, -11.25)
  line L691 (4.8182, -11.25) -> (4.8182, -10.75)
  line L692 (2.6364, -12.75) -> (5.3636, -12.75)
  line L693 (5.3636, -12.75) -> (5.3636, -13.25)
  line L694 (5.3636, -13.25) -> (2.6364, -13.25)
  line L695 (2.6364, -13.25) -> (2.6364, -12.75)
  line L696 (1, -10.75) -> (3.1818, -10.75)
  line L697 (3.1818, -10.75) -> (3.1818, -11.25)
  line L698 (3.1818, -11.25) -> (1, -11.25)
  line L699 (1, -11.25) -> (1, -10.75)
  line L700 (1, -12) -> (7, -12) construction
  line L701 (7, -12) -> (1, -12) construction
  line L702 (4.8182, -6.75) -> (7, -6.75)
  line L703 (7, -6.75) -> (7, -7.25)
  line L704 (7, -7.25) -> (4.8182, -7.25)
  line L705 (4.8182, -7.25) -> (4.8182, -6.75)
  line L706 (2.6364, -8.75) -> (5.3636, -8.75)
  line L707 (5.3636, -8.75) -> (5.3636, -9.25)
  line L708 (5.3636, -9.25) -> (2.6364, -9.25)
  line L709 (2.6364, -9.25) -> (2.6364, -8.75)
  line L710 (1, -6.75) -> (3.1818, -6.75)
  line L711 (3.1818, -6.75) -> (3.1818, -7.25)
  line L712 (3.1818, -7.25) -> (1, -7.25)
  line L713 (1, -7.25) -> (1, -6.75)
  line L714 (1, -8) -> (7, -8) construction
  line L715 (7, -8) -> (1, -8) construction
  line L716 (4.8182, -2.75) -> (7, -2.75)
  line L717 (7, -2.75) -> (7, -3.25)
  line L718 (7, -3.25) -> (4.8182, -3.25)
  line L719 (4.8182, -3.25) -> (4.8182, -2.75)
  line L720 (2.6364, -4.75) -> (5.3636, -4.75)
  line L721 (5.3636, -4.75) -> (5.3636, -5.25)
  line L722 (5.3636, -5.25) -> (2.6364, -5.25)
  line L723 (2.6364, -5.25) -> (2.6364, -4.75)
  line L724 (1, -2.75) -> (3.1818, -2.75)
  line L725 (3.1818, -2.75) -> (3.1818, -3.25)
  line L726 (3.1818, -3.25) -> (1, -3.25)
  line L727 (1, -3.25) -> (1, -2.75)
  line L728 (1, -4) -> (7, -4) construction
  line L729 (7, -4) -> (1, -4) construction
  line L730 (4.8182, 13.25) -> (7, 13.25)
  line L731 (7, 13.25) -> (7, 12.75)
  line L732 (7, 12.75) -> (4.8182, 12.75)
  line L733 (4.8182, 12.75) -> (4.8182, 13.25)
  line L734 (2.6364, 11.25) -> (5.3636, 11.25)
  line L735 (5.3636, 11.25) -> (5.3636, 10.75)
  line L736 (5.3636, 10.75) -> (2.6364, 10.75)
  line L737 (2.6364, 10.75) -> (2.6364, 11.25)
  line L738 (1, 13.25) -> (3.1818, 13.25)
  line L739 (3.1818, 13.25) -> (3.1818, 12.75)
  line L740 (3.1818, 12.75) -> (1, 12.75)
  line L741 (1, 12.75) -> (1, 13.25)
  line L742 (1, 12) -> (7, 12) construction
  line L743 (7, 12) -> (1, 12) construction
  line L744 (4.8182, 9.25) -> (7, 9.25)
  line L745 (7, 9.25) -> (7, 8.75)
  line L746 (7, 8.75) -> (4.8182, 8.75)
  line L747 (4.8182, 8.75) -> (4.8182, 9.25)
  line L748 (2.6364, 7.25) -> (5.3636, 7.25)
  line L749 (5.3636, 7.25) -> (5.3636, 6.75)
  line L750 (5.3636, 6.75) -> (2.6364, 6.75)
  line L751 (2.6364, 6.75) -> (2.6364, 7.25)
  line L752 (1, 9.25) -> (3.1818, 9.25)
  line L753 (3.1818, 9.25) -> (3.1818, 8.75)
  line L754 (3.1818, 8.75) -> (1, 8.75)
  line L755 (1, 8.75) -> (1, 9.25)
  line L756 (1, 8) -> (7, 8) construction
  line L757 (7, 8) -> (1, 8) construction
  line L758 (4.8182, 5.25) -> (7, 5.25)
  line L759 (7, 5.25) -> (7, 4.75)
  line L760 (7, 4.75) -> (4.8182, 4.75)
  line L761 (4.8182, 4.75) -> (4.8182, 5.25)
  line L762 (2.6364, 3.25) -> (5.3636, 3.25)
  line L763 (5.3636, 3.25) -> (5.3636, 2.75)
  line L764 (5.3636, 2.75) -> (2.6364, 2.75)
  line L765 (2.6364, 2.75) -> (2.6364, 3.25)
  line L766 (1, 5.25) -> (3.1818, 5.25)
  line L767 (3.1818, 5.25) -> (3.1818, 4.75)
  line L768 (3.1818, 4.75) -> (1, 4.75)
  line L769 (1, 4.75) -> (1, 5.25)
  line L770 (1, 4) -> (7, 4) construction
  line L771 (7, 4) -> (1, 4) construction
  line L772 (4.8182, 1.25) -> (7, 1.25)
  line L773 (7, 1.25) -> (7, 0.75)
  line L774 (7, 0.75) -> (4.8182, 0.75)
  line L775 (4.8182, 0.75) -> (4.8182, 1.25)
  line L776 (2.6364, -0.75) -> (5.3636, -0.75)
  line L777 (5.3636, -0.75) -> (5.3636, -1.25)
  line L778 (5.3636, -1.25) -> (2.6364, -1.25)
  line L779 (2.6364, -1.25) -> (2.6364, -0.75)
  line L780 (1, 1.25) -> (3.1818, 1.25)
  line L781 (3.1818, 1.25) -> (3.1818, 0.75)
  line L782 (3.1818, 0.75) -> (1, 0.75)